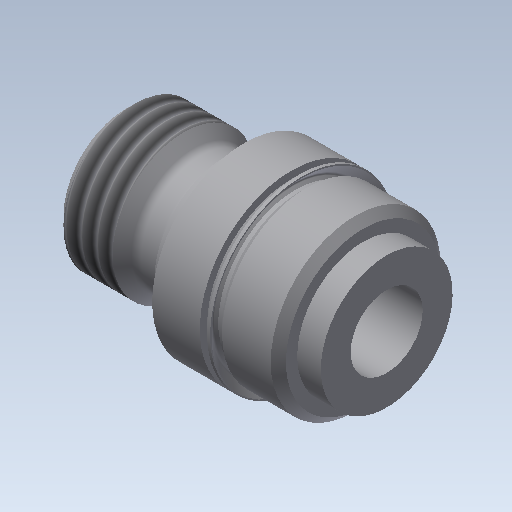
# Autodesk Inventor part: 01000-0_rod_guide
Saved by Autodesk Inventor 2020 (Build 240168000, 168)
## iProperties
Created: 2020-01-07
Part Number: 01000-0_rod_guide
Material: Generic
Catalog Web Link: www.cadenas.de
Description: Rod Guide-Original Line - Standard Air Cylinders
Vendor: BIMBA
Document SubType Name: Modeling
Designer: psadmin
Manufacturer: BIMBA
Mass: 1.13414 g
Surface Area: 11.0116 cm^2
Volume: 1.13414 cm^3
Density: 1 g/cm^3
Appearance: PSOLRGB-211-211-211
Category: PARTsolutions
Company: BIMBA
PSOL_IDENT_0: {$CADENAS_DATA\23d-libs\bimba\bimba_brand\bimba_imperial\bimba_full_line\original_line_cylinders\sta
PSOL_IDENT_1: ndard_air_cylinders\rod_guide.prj},249 {VTYP=3D},{NB=01000-0_rod_guide},{LINA=01000-0_rod_guide},{NN=
PSOL_IDENT_2: Rod Guide},{DATE=23.12.2019 10:36:48},{GEOMDATE=15.10.2019 12:06:01},{VERSION=},{LINEID=20},{WBVAR=M
PSOL_IDENT_3: NT,ACTING,NR,K,Q,T1,T2,T3,T4,MB,TRIM,CUSH,RODTRANS},{WBNUMERIC=MB,TRIM,CUSH,RODTRANS}  {NB=01000-0_r
PSOL_IDENT_4: od_guide},{LINA=01000-0_rod_guide},{KT=DUMMY},{PN=01000},{BORE=0.43750000},{BOREPN=01},{MNT=},{MNTAL
PSOL_IDENT_5: G='' , 'Front Nose' , 'BF' , 'Front Block' , 'BFT' , 'Front Trunnion'},{ACTING=},{ACTINGALG= '' , 'S
PSOL_IDENT_6: ingle Acting' , 'R' , 'Reverse/Double Acting' },{NR=},{NRALG= '' , 'Without Non-rotating Rod' , 'NR'
PSOL_IDENT_7: , 'With Non-rotating Rod' },{K=},{Q=},{QALG= '' , 'Without Side Ported Rear Head' , 'Q' , 'With Sid
PSOL_IDENT_8: e Ported Rear Head' },{T1=},{T2=},{T3=},{T4=},{MB=0},{A1=0.6880},{A1N=0.6880},{A1P=1.1880},{A1B=1.18
PSOL_IDENT_9: 80},{A2=0.3130},{A2N=0.3130},{A2P=0.3750},{A3=0.1250},{A3N=0.1250},{A3P=0.6250},{A4=0.2500},{A4N=0.2
PSOL_IDENT_10: 500},{A4P=0.1880},{A5=0.0200},{A6=0.0620},{A6N=0.0620},{A6P=0.0000},{A7=0.1880},{A7N=0.1880},{A7P=0.
PSOL_IDENT_11: 5940},{A8=0.0200},{A8N=0.0200},{A8NR=0.0200},{D1=0.4840},{D1N=0.4840},{D1P=0.7380},{D1B=0.0000},{D2=
PSOL_IDENT_12: 0.4465},{D3=0.3470},{D3N=0.3470},{D3P=0.0000},{D4=0.2220},{D4N=0.2220},{D4P=0.2820},{D4NR=0.2820},{D
PSOL_IDENT_13: 5=0.1895},{D5N=0.1895},{D5NR=0.1895},{C1=0.000},{C2=0.0200},{C2N=0.0200},{C2P=0.0200},{C3=0.0000},{C
PSOL_IDENT_14: 3N=0.0000},{C3P=0.0000},{C4=0.0000},{C4N=0.0000},{C4P=0.0000},{NDM=0.3750},{NDMN=0.3750},{NDMP=0.437
PSOL_IDENT_15: 5},{TAB=UNF},{D6=0.3725},{D6N=0.3725},{D6P=0.4350},{A9=0.0500},{A9N=0.0500},{A9P=0.0475},{D7=0.3100}
PSOL_IDENT_16: ,{D7N=0.3100},{D7P=0.3600},{A10=0.0655},{A10N=0.0655},{A10P=0.0775},{R1=0.0265},{R1N=0.0265},{R1P=0.
PSOL_IDENT_17: 0315},{D8=0.0000},{D9=0.0000},{D10=0.0000},{A11=0.0000},{A12=0.0000},{A13=0.0000},{A14=0.4680},{A14N=
PSOL_IDENT_18: 0.4680},{A14B=0.4690},{D11=0.0000},{D11N=0.0000},{NDM2=0.1900},{NDM2N=0.1900},{NDM2DP=0.0000},{THREA
PSOL_IDENT_19: D=0},{HEX=0.1920},{HEXN=0.1920},{S1=0.7500},{B1=0.1275},{B2=0.3120},{B22=0.4380},{DB=0.3020},{B3=0.2
PSOL_IDENT_20: 200},{B4=0.4380},{X1=0.0620},{X2=0.4345},{NDM3=0.1640},{NDM4=0.1640},{NDM4DP=0.2500},{DD=0.7500},{CB=
PSOL_IDENT_21: 0.0000},{CBDP=0.0000},{PORT=1},{XT=0.3120},{XTX=0.3120},{XT1=0.3740},{XT2=0.2500},{NDMH=0.0000},{OD=
PSOL_IDENT_22: 0.4840},{ID=0.4465},{G=0.0000},{PNUT=0.2630},{TRIM=0},{C11=0.0000},{C22=0.0000},{C33=0.0000},{C44=0.
PSOL_IDENT_23: 0000},{C55=0.0000},{CD1=0.0000},{CD2=0.0000},{CD3=0.0000},{CNDM3=0.0000},{CTAB3=0.0000},{CUSH=0},{XX=
PSOL_IDENT_24: 0.43800},{LCD=0.0000},{RODTRANS=0.00000}
NN: Rod Guide
NT: Original Line - Standard Air Cylinders
NB: 01000-0_rod_guide
NBSYN: $PN.-$RODTRANS._rod_guide
LINA: 01000-0_rod_guide
BORE: 0
BOREPN: 01
MNT: Front Nose
MNTALG: '' , 'Front Nose' , 'BF' , 'Front Block' , 'BFT' , 'Front Trunnion'
ACTING: Single Acting
NR: Without Non-rotating Rod
K: Standard
Q: Without Side Ported Rear Head
T1: without T1
T2: without T2
T3: without T3
T4: without T4
MB: 0
A1N: 0.688
A1P: 1.188
A1B: 1.188
A2N: 0.313
A2P: 0.375
A3N: 0.125
A3P: 0.625
A4N: 0.25
A4P: 0.188
A5: 0.02
A6N: 0.062
A6P: 0
A7N: 0.188
A7P: 0.594
A8N: 0.02
A8NR: 0.02
D1N: 0.484
D1P: 0.738
D1B: 0
D2: 0.4465
D3N: 0.347
D3P: 0
D4N: 0.222
D4P: 0.282
D4NR: 0.282
D5N: 0.1895
D5NR: 0.1895
C1: 0
C2N: 0.02
C2P: 0.02
C3N: 0
C3P: 0
C4N: 0
C4P: 0
NDMN: 0.375
NDMP: 0.4375
TAB: UNF
D6N: 0.3725
D6P: 0.435
A9N: 0.05
A9P: 0.0475
D7N: 0.31
D7P: 0.36
A10N: 0.0655
A10P: 0.0775
R1N: 0.0265
R1P: 0.0315
D8: 0
D9: 0
D10: 0
A11: 0
A12: 0
A13: 0
A14N: 0.468
A14B: 0.469
D11N: 0
NDM2N: 0.19
NDM2DP: 0
HEXN: 0.192
S1: 0.75
B1: 0.1275
B2: 0.312
B22: 0.438
DB: 0.302
B3: 0.22
B4: 0.438
X1: 0.062
X2: 0.4345
NDM3: 0.164
NDM4: 0.164
NDM4DP: 0.25
DD: 0.75
CB: 0
CBDP: 0
XTX: 0.312
XT1: 0.374
XT2: 0.25
NDMH: 0
TRIM: 0
C11: 0
C22: 0
C33: 0
C44: 0
C55: 0
CD1: 0
CD2: 0
CD3: 0
CNDM3: 0
CTAB3: 0.0000
CUSH: 0
LCD: 0
RODTRANS: 0
SUPPLIER: BIMBA
ARTICLENO: 01000-0_rod_guide
BOMINFO: 01000-0_rod_guide
CREATOR: CADENAS GmbH
d13: 0.000 in
d14: 0.000 in
d15: 0.000 in
d16: 0.000 in
d17: 0.000 in
d18: 0.000 in
Title: 01000-0_rod_guide
Author: Cadenas PARTsolutions
Comments: Original Line - Standard Air Cylinders
Autodesk Inventor part; units mm, degrees
sketch "Sketch_2" plane through (0, 0, 0) normal (0, 0, 1) x (1, 0, 0)
  line L0 (7.9502, 0) -> (0, 0)
  line L1 (0, 0) -> (0, 4.1326)
  line L2 (0, 4.1326) -> (0.6299, 4.7625)
  line L3 (0.6299, 4.7625) -> (3.9106, 4.7625)
  line L4 (3.9106, 4.7625) -> (4.5411, 4.1336)
  arc A0 (4.5411, 4.1336) -> (5.0165, 3.937) centre (5.0165, 4.6101) ccw
  line L5 (5.0165, 3.937) -> (6.0071, 3.937)
  arc A1 (6.0071, 3.937) -> (6.6802, 4.6101) centre (6.0071, 4.6101) ccw
  line L6 (6.6802, 4.6101) -> (6.6802, 4.7307)
  line L7 (6.6802, 4.7307) -> (7.9502, 4.7307)
  line L8 (7.9502, 4.7307) -> (7.9502, 0)
  line L9 (7.9502, 0) -> (0, 0)
  constraints: 20 end point, 4 point on circle, 2 centre point
revolve "Revolution1" add sketch "Sketch_2" angle 360 about axis through (7.9502, 0, 0) along (1, 0, 0)
thread "Thread1" size "3/8-24 UNF" class "2A" standard "ANSI Unified Screw Threads" full length
sketch "Sketch_3" plane through (0, 0, 0) normal (0, 0, 1) x (1, 0, 0)
  line L0 (15.9004, 0) -> (7.9502, 0)
  line L1 (7.9502, 0) -> (7.9502, 6.1468)
  line L2 (7.9502, 6.1468) -> (11.1252, 6.1468)
  line L3 (11.1252, 6.1468) -> (11.1252, 5.1626)
  line L4 (11.1252, 5.1626) -> (11.6332, 5.1626)
  line L5 (11.6332, 5.1626) -> (12.1412, 5.6706)
  line L6 (12.1412, 5.6706) -> (15.3924, 5.6706)
  line L7 (15.3924, 5.6706) -> (15.9004, 5.1626)
  line L8 (15.9004, 5.1626) -> (15.9004, 0)
  line L9 (15.9004, 0) -> (7.9502, 0)
  constraints: 20 end point
revolve "Revolution2" add sketch "Sketch_3" angle 360 about axis through (15.9004, 0, 0) along (1, 0, 0)
sketch "Sketch_4" plane through (0, 0, 0) normal (0, 0, 1) x (1, 0, 0)
  line L0 (17.4752, 0) -> (15.9004, 0)
  line L1 (15.9004, 0) -> (15.9004, 4.4069)
  line L2 (15.9004, 4.4069) -> (17.4752, 4.4069)
  line L3 (17.4752, 4.4069) -> (17.4752, 0)
  line L4 (17.4752, 0) -> (15.9004, 0)
  constraints: 10 end point
revolve "Revolution3" add sketch "Sketch_4" angle 360 about axis through (17.4752, 0, 0) along (1, 0, 0)
sketch "Sketch4" plane through (0, 0, 0) normal (-1, 0, 0) x (0, 0, 1)
  point P0 (0, 0)
hole "Hole1" at (0, 0, 0) direction (1, 0, 0) diameter 4.8133 depth 17.4752 countersink diameter 5.8293 countersink angle 90
sketch "Sketch_47" plane through (0, 0, 0) normal (0, 0, 1) x (1, 0, 0)
  line L0 (11.6332, 0) -> (11.1252, 0)
  line L1 (11.1252, 5.6603) -> (11.1252, 4.9085)
  line L2 (11.1252, 4.9085) -> (11.6332, 4.9085)
  line L3 (11.6332, 4.9085) -> (11.6332, 5.1626)
  line L4 (11.6332, 5.1626) -> (11.3792, 5.1626)
  line L5 (11.3792, 5.1626) -> (11.2368, 5.305)
  arc A0 (11.2368, 5.4846) -> (11.2368, 5.305) centre (11.3266, 5.3948) ccw
  line L6 (11.2368, 5.4846) -> (11.8149, 6.0626)
  line L7 (11.8149, 6.0626) -> (11.8149, 6.1468)
  line L8 (11.8149, 6.1468) -> (11.6117, 6.1468)
  line L9 (11.6117, 6.1468) -> (11.1252, 5.6603)
  constraints: 20 end point, 2 point on circle, 1 centre point
revolve "Revolution4" add sketch "Sketch_47" angle 360 about axis through (11.6332, 0, 0) along (1, 0, 0)
ref_plane "dp1_XY" through (7.9502, 4.7307, 0) normal (0, 0, 1) x (1, 0, 0)
ref_plane "dp1_YZ" through (7.9502, 4.7307, 0) normal (1, 0, 0) x (0, 1, 0)
ref_plane "dp1_ZX" through (7.9502, 4.7307, 0) normal (0, 1, 0) x (0, 0, 1)
ref_plane "dp2_XY" through (7.9502, -4.7307, 0) normal (0, 0, 1) x (1, 0, 0)
ref_plane "dp2_YZ" through (7.9502, -4.7307, 0) normal (1, 0, 0) x (0, 1, 0)
ref_plane "dp2_ZX" through (7.9502, -4.7307, 0) normal (0, 1, 0) x (0, 0, 1)
ref_plane "hh_XY" through (0, 4.7625, 0) normal (0, 0, 1) x (1, 0, 0)
ref_plane "hh_YZ" through (0, 4.7625, 0) normal (1, 0, 0) x (0, 1, 0)
ref_plane "hh_ZX" through (0, 4.7625, 0) normal (0, 1, 0) x (0, 0, 1)
ref_plane "rod_guide_XY" through (0, 0, 0) normal (1, 0, 0) x (0, 0, -1)
ref_plane "rod_guide_YZ" through (0, 0, 0) normal (0, 0, -1) x (0, 1, 0)
ref_plane "rod_guide_ZX" through (0, 0, 0) normal (0, 1, 0) x (1, 0, 0)
ref_plane "s1_XY" through (6.6802, 0, 0) normal (0, 0, 1) x (1, 0, 0)
ref_plane "s1_YZ" through (6.6802, 0, 0) normal (1, 0, 0) x (0, 1, 0)
ref_plane "s1_ZX" through (6.6802, 0, 0) normal (0, 1, 0) x (0, 0, 1)
ref_plane "s2_XY" through (7.9502, 0, 0) normal (0, 0, 1) x (1, 0, 0)
ref_plane "s2_YZ" through (7.9502, 0, 0) normal (1, 0, 0) x (0, 1, 0)
ref_plane "s2_ZX" through (7.9502, 0, 0) normal (0, 1, 0) x (0, 0, 1)
ref_plane "t1_XY" through (7.9502, 0, 0) normal (1, 0, 0) x (0, 0, -1)
ref_plane "t1_YZ" through (7.9502, 0, 0) normal (0, 0, -1) x (0, 1, 0)
ref_plane "t1_ZX" through (7.9502, 0, 0) normal (0, 1, 0) x (1, 0, 0)
ref_plane "t111_XY" through (7.9502, 0, 0) normal (1, 0, 0) x (0, 0, -1)
ref_plane "t111_YZ" through (7.9502, 0, 0) normal (0, 0, -1) x (0, 1, 0)
ref_plane "t111_ZX" through (7.9502, 0, 0) normal (0, 1, 0) x (1, 0, 0)
ref_plane "to_foot_bracket_XY" through (7.9502, 0, 0) normal (1, 0, 0) x (0, 0, -1)
ref_plane "to_foot_bracket_YZ" through (7.9502, 0, 0) normal (0, 0, -1) x (0, 1, 0)
ref_plane "to_foot_bracket_ZX" through (7.9502, 0, 0) normal (0, 1, 0) x (1, 0, 0)
ref_plane "to_nut_XY" through (6.6802, 0, 0) normal (1, 0, 0) x (0, 0, -1)
ref_plane "to_nut_YZ" through (6.6802, 0, 0) normal (0, 0, -1) x (0, 1, 0)
ref_plane "to_nut_ZX" through (6.6802, 0, 0) normal (0, 1, 0) x (1, 0, 0)
ref_plane "to_rod_XY" through (0, 0, 0) normal (1, 0, 0) x (0, 0, -1)
ref_plane "to_rod_YZ" through (0, 0, 0) normal (0, 0, -1) x (0, 1, 0)
ref_plane "to_rod_ZX" through (0, 0, 0) normal (0, 1, 0) x (1, 0, 0)
ref_plane "to_screw_XY" through (5.588, 0, 0) normal (0, 1, 0) x (1, 0, 0)
ref_plane "to_screw_YZ" through (5.588, 0, 0) normal (1, 0, 0) x (0, 0, -1)
ref_plane "to_screw_ZX" through (5.588, 0, 0) normal (0, 0, -1) x (0, 1, 0)
ref_plane "to_trunnion_brackets_XY" through (7.9248, 0, 0) normal (0, 1, 0) x (1, 0, 0)
ref_plane "to_trunnion_brackets_YZ" through (7.9248, 0, 0) normal (1, 0, 0) x (0, 0, -1)
ref_plane "to_trunnion_brackets_ZX" through (7.9248, 0, 0) normal (0, 0, -1) x (0, 1, 0)
ref_plane "to_trunnion_brackets1_XY" through (7.9248, 9.525, 0) normal (0, 1, 0) x (1, 0, 0)
ref_plane "to_trunnion_brackets1_YZ" through (7.9248, 9.525, 0) normal (1, 0, 0) x (0, 0, -1)
ref_plane "to_trunnion_brackets1_ZX" through (7.9248, 9.525, 0) normal (0, 0, -1) x (0, 1, 0)
ref_plane "to_trunnion_brackets2_XY" through (7.9248, -9.525, 0) normal (0, 1, 0) x (1, 0, 0)
ref_plane "to_trunnion_brackets2_YZ" through (7.9248, -9.525, 0) normal (1, 0, 0) x (0, 0, -1)
ref_plane "to_trunnion_brackets2_ZX" through (7.9248, -9.525, 0) normal (0, 0, -1) x (0, 1, 0)
ref_plane "to_tube_XY" through (11.6332, 0, 0) normal (1, 0, 0) x (0, 0, -1)
ref_plane "to_tube_YZ" through (11.6332, 0, 0) normal (0, 0, -1) x (0, 1, 0)
ref_plane "to_tube_ZX" through (11.6332, 0, 0) normal (0, 1, 0) x (1, 0, 0)
body "Solid1"
